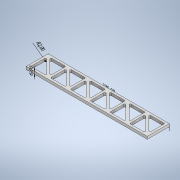
# Autodesk Inventor part: Część13
Saved by Autodesk Inventor 2021 (Build 250183000, 183)
## iProperties
Created: 2023-10-06
Part Number: Część13
Material: Ogólny
Document SubType Name: Modeling
Designer: Jakub
Density: 1 g/cm^3
Appearance: Domyślna
Author: Jakub
Autodesk Inventor part; units mm, degrees
ref_plane "YZ Plane" through (0, 0, 0) normal (1, 0, 0) x (0, 1, 0)
ref_plane "XZ Plane" through (0, 0, 0) normal (0, 1, 0) x (-1, 0, 0)
ref_plane "XY Plane" through (0, 0, 0) normal (0, 0, 1) x (1, 0, 0)
sketch "Szkic1" plane through (0, 0, 0) normal (0, 1, 0) x (-1, 0, 0)
  line L0 (0, 0) -> (0, -50)
  line L1 (0, -50) -> (-50, -50)
  line L2 (-50, -50) -> (-50, 0)
  line L3 (0, 0) -> (-50, 0)
  line L4 (-5, -15) -> (0, -15)
  line L5 (-15, 0) -> (-15, -5)
  line L6 (-15, -5) -> (-5, -5)
  line L7 (-5, -5) -> (-5, -15)
  line L8 (-40, -50) -> (-40, -45)
  line L9 (-40, -45) -> (-45, -45)
  line L10 (-45, -45) -> (-45, 0)
  line L11 (-40, -45) -> (0, -45)
  line L12 (-5, -15) -> (-5, -50)
  line L13 (-15, -5) -> (-50, -5)
  line L14 (0, -50) -> (-50, 0)
  line L15 (-25, -25) -> (-26.7678, -26.7678)
  line L16 (-26.7678, -26.7678) -> (-23.2322, -23.2322)
  line L17 (-23.2322, -23.2322) -> (0, -46.4645)
  line L18 (-23.2322, -23.2322) -> (-46.4645, 0)
  line L19 (-26.7678, -26.7678) -> (-50, -3.5355)
  line L20 (-26.7678, -26.7678) -> (-3.5355, -50)
  point P0 (-45, -8.5355)
  point P1 (-8.5355, -45)
  point P2 (-5, -41.4645)
  point P3 (-41.4645, -5)
  dimension "d0" = 50
  dimension "d1" = 50
  dimension "d2" = 5
  dimension "d3" = 5
  dimension "d4" = 5
  dimension "d5" = 2.5
  dimension "d6" = 5
  constraints: 42 end point, 15 point on line, 11 perpendicular, 2 vertical, 1 horizontal, 1 midpoint, 1 parallel
  measures "d0" distance of L0.start L0.end
  measures "d1" distance of L0.end L1.end
  measures "d2" distance of L5.start L5.end
  measures "d3" distance of L8.start L8.end
  measures "d4" distance of L8.end L9.end
  measures "d5" distance of L15.start L15.end
  measures "d6" distance of L15.end L16.end
extrude "Wyciągnięcie proste1" add sketch "Szkic1" along normal blind 6 contours L0 L4 L7 L6 L5 L3 | L0 L11 L17 L12 L4 | L5 L13 L18 L10 L3 | L0 L17 L11 | L10 L18 L3 | L0 L14 L11 L17 | L11 L12 L17 | L12 L14 L16 L17 | L18 L10 L14 L3 | L18 L13 L10 | L18 L16 L14 L13 | L1 L20 L12 L14 | L12 L20 L11 | L11 L20 L15 L14 | L14 L13 L19 L2 | L14 L15 L19 L10 | L10 L19 L13 | L1 L12 L20 | L20 L12 L1 L8 L11 | L19 L13 L2 | L10 L9 L8 L1 L2 L13 L19
fillet "Zaokrąglenie1" radius 2 6 edges at (8.5355, 3, -45) (5, 3, -41.4645) (45, 3, -8.5355) (41.4645, 3, -5) (45, 3, -45) (5, 3, -5)
pattern_linear "Szyk prostokątny1" count 6 spacing 45 along (1, 0, 0) of "Wyciągnięcie proste1"
fillet "Zaokrąglenie2" radius 2 25 edges at (53.5355, 3, -45) (98.5355, 3, -45) (143.5355, 3, -45) (188.5355, 3, -45) (233.5355, 3, -45) (230, 3, -5) (185, 3, -5) (140, 3, -5) (95, 3, -5) (50, 3, -5) (86.4645, 3, -5) (131.4645, 3, -5) (176.4645, 3, -5) (221.4645, 3, -5) (266.4645, 3, -5) (270, 3, -45) (225, 3, -45) (180, 3, -45) (135, 3, -45) (90, 3, -45) (50, 3, -41.4645) (95, 3, -41.4645) (140, 3, -41.4645) (185, 3, -41.4645) (230, 3, -41.4645)
fillet "Zaokrąglenie3" radius 2 5 edges at (270, 3, -8.5355) (225, 3, -8.5355) (180, 3, -8.5355) (135, 3, -8.5355) (90, 3, -8.5355)
